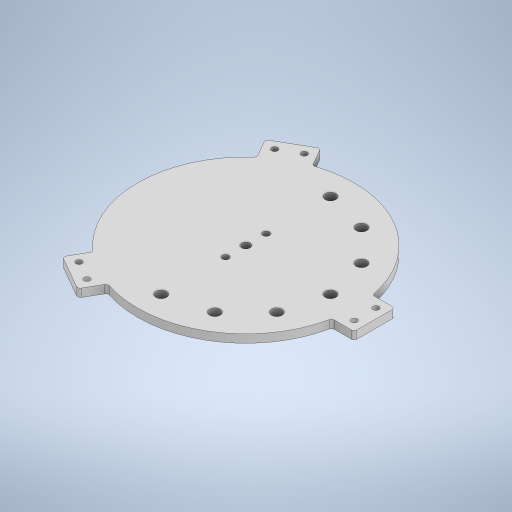
# Autodesk Inventor part: SkimmerLid
Saved by Autodesk Inventor 2023.2 (Build 272271000, 271)
## iProperties
Created: 2023-02-16
Part Number: SkimmerLid
Material: Generic
Document SubType Name: Modeling
Designer: atrus
Density: 1 g/cm^3
Appearance: Default
Author: atrus
Autodesk Inventor part; units mm, degrees
ref_plane "YZ Plane" through (0, 0, 0) normal (1, 0, 0) x (0, 1, 0)
ref_plane "XZ Plane" through (0, 0, 0) normal (0, 1, 0) x (-1, 0, 0)
ref_plane "XY Plane" through (0, 0, 0) normal (0, 0, 1) x (1, 0, 0)
sketch "Sketch1" plane through (0, 0, 0) normal (0, 1, 0) x (-1, 0, 0)
  line L0 (0, 80) -> (0, 62.5) construction
  circle A0 centre (0, 62.5) radius 4
  line L1 (0, 62.5) -> (0, 0) construction
  circle A1 centre (-31.25, 54.1266) radius 4
  circle A2 centre (-54.1266, 31.25) radius 4
  circle A3 centre (-62.5, 0) radius 4
  circle A4 centre (-54.1266, -31.25) radius 4
  circle A5 centre (-31.25, -54.1266) radius 4
  circle A6 centre (0, -62.5) radius 4
  circle A7 centre (0, 0) radius 3.175
  line L2 (-78.5812, -15) -> (-95, -15)
  line L3 (-95, -15) -> (-95, 15)
  line L4 (-95, 15) -> (-78.5812, 15)
  line L5 (52.281, -60.5533) -> (60.4904, -74.7724)
  line L6 (60.4904, -74.7724) -> (34.5096, -89.7724)
  line L7 (34.5096, -89.7724) -> (26.3002, -75.5533)
  line L8 (26.3002, 75.5533) -> (34.5096, 89.7724)
  line L9 (34.5096, 89.7724) -> (60.4904, 74.7724)
  line L10 (60.4904, 74.7724) -> (52.281, 60.5533)
  arc A8 (52.281, -60.5533) -> (52.281, 60.5533) centre (0, 0) ccw
  arc A9 (26.3002, 75.5533) -> (-78.5812, 15) centre (0, 0) ccw
  arc A10 (-78.5812, -15) -> (26.3002, -75.5533) centre (0, 0) ccw
  point P0 (80, 0)
  dimension "d2" = 8
  dimension "d5" = 180
  dimension "d7" = 6.35
  dimension "d10" = 62.5
  dimension "d12" = 95
  dimension "d13" = 30
  dimension "d16" = 360
  dimension "d18" = 80
  constraints: 22 end point, 11 centre point, 8 point on circle, 4 coincident, 2 parallel, 1 collinear, 1 horizontal, 1 perpendicular, 1 vertical, 35 other
  measures "d2" diameter of A0
  measures "d7" diameter of A7
  measures "d10" distance of point (0, 0) L0.end
  measures "d12" distance from line of L3 point (0, 0)
  measures "d13" distance of L2.end L3.end
  measures "d18" distance of L1.end point (80, 0)
extrude "Extrusion1" add sketch "Sketch1" along normal blind 6
sketch "Sketch3" plane through (0, 6, 0) normal (0, 1, 0) x (1, 0, 0)
  line L0 (95, 15) -> (78.5812, 15) projected
  line L1 (78.5812, -15) -> (95, -15) projected
  line L2 (95, -15) -> (95, 15) projected
  point P0 (0, 0)
  point P1 (88, 8)
  point P2 (88, -8)
  point P3 (86.7906, -15)
  point P4 (-50.9282, 72.2102)
  point P5 (-37.0718, 80.2102)
  point P6 (-37.0718, -80.2102)
  point P7 (-50.9282, -72.2102)
  dimension "d19" = 7
  dimension "d20" = 7
  dimension "d21" = 7
  dimension "d24" = 360
  constraints: 1 midpoint, 1 vertical alignment, 7 other
  measures "d19" distance from line of point (88, 8) L0
  measures "d20" vertical distance of point (86.791, -15) point (88, -8)
  measures "d21" distance from line of L2 point (88, -8)
hole "Hole1" at (88, 6, -8) at (88, 6, 8) at (-50.9282, 6, -72.2102) at (-37.0718, 6, -80.2102) at (-37.0718, 6, 80.2102) at (-50.9282, 6, 72.2102) direction (0, -1, 0) diameter 4.5 end through all clearance for "Flat Head Machine Screw" size "M4" standard "Ansi Metric M Profile"
sketch "Sketch4" plane through (0, 6, 0) normal (0, 1, 0) x (1, 0, 0)
  circle A0 centre (0, 15) radius 2.5
  circle A1 centre (0, -15) radius 2.5
  circle A2 centre (0, 0) radius 3.175 construction
  line L0 (0, 0) -> (8.7984, 0) construction
  dimension "d33" = 5
  dimension "d34" = 15
  constraints: 2 centre point, 2 end point, 1 equal radius, 1 horizontal, 1 symmetric about line
  measures "d33" diameter of A0
  measures "d34" distance of A0.centre point (0, 0)
extrude "Extrusion2" cut sketch "Sketch4" against normal blind 6
fillet "Fillet1" radius 2 12 edges at (-52.281, 3, 60.5533) (-60.4904, 3, 74.7724) (-34.5096, 3, 89.7724) (-26.3002, 3, 75.5533) (78.5812, 3, 15) (95, 3, 15) (95, 3, -15) (78.5812, 3, -15) (-26.3002, 3, -75.5533) (-34.5096, 3, -89.7724) (-52.281, 3, -60.5533) (-60.4904, 3, -74.7724)
body "Solid1"
